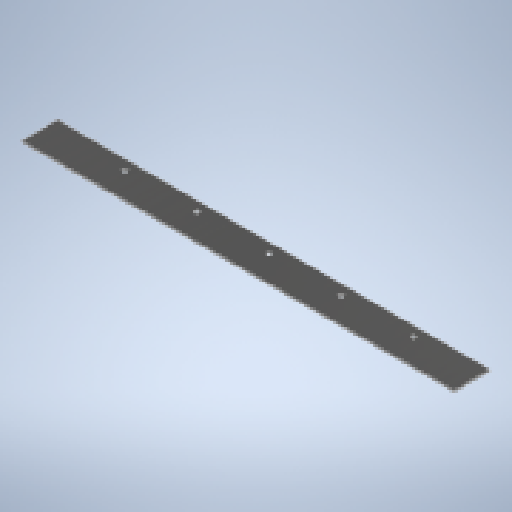
# Autodesk Inventor part: HCMUTE-CDT23-BTC-VND
Saved by Autodesk Inventor 2023 (Build 270158000, 158)
## iProperties
Created: 2023-11-27
Part Number: HCMUTE-CDT23-BTC-VND
Material: PMMA Plastic
Document SubType Name: Sheet Metal
Designer: havie
Density: 1.188 g/cm^3
Sheet Metal Rule: Default_mm
Appearance: Dark Gray
Author: havie
Autodesk Inventor part; units mm, degrees
ref_plane "YZ Plane" through (0, 0, 0) normal (1, 0, 0) x (0, 1, 0)
ref_plane "XZ Plane" through (0, 0, 0) normal (0, 1, 0) x (-1, 0, 0)
ref_plane "XY Plane" through (0, 0, 0) normal (0, 0, 1) x (1, 0, 0)
sketch "Sketch1" plane through (0, 0, 0) normal (0, 1, 0) x (-1, 0, 0)
  line L0 (-300, 25) -> (300, 25)
  line L1 (300, 25) -> (300, -25)
  line L2 (300, -25) -> (-300, -25)
  line L3 (-300, -25) -> (-300, 25)
  line L4 (-300, 25) -> (300, -25) construction
  line L5 (300, 25) -> (-300, -25) construction
  point P0 (0, 0)
  dimension "d0" = 600
  dimension "d1" = 50
  measures "d0" distance of L1.end L2.end
  measures "d1" distance of L2.end L0.start
extrude "Plate1" add sketch "Sketch1" along normal mid plane 2
sketch "Sketch2" plane through (0, -1, 0) normal (0, -1, 0) x (1, 0, 0)
  circle A0 centre (-192.5, -11) radius 2.5 projected
  circle A1 centre (-92.5, -11) radius 2.5 projected
  circle A2 centre (7.5, -11) radius 2.5 projected
  line L0 (300, 25) -> (-300, 25) projected
  line L1 (-300, 25) -> (-300, -25) projected
  line L2 (-300, -25) -> (300, -25) projected
  line L3 (300, -25) -> (300, 25) projected
  circle A3 centre (107.5, -11) radius 2.5 projected
  circle A4 centre (207.5, -11) radius 2.5 projected
  point P0 (0, 0)
  constraints: 5 coincident
hole "Hole1" at (-192.5, -1, -11) at (-92.5, -1, -11) at (7.5, -1, -11) at (107.5, -1, -11) at (207.5, -1, -11) direction (0, 1, 0) diameter 6 end through all
equation "\"d8\" = Thickness"
equation "\"d2\" = Thickness"
equation "\"BendRadius\" = Thickness"
equation "\"BendReliefWidth\" = Thickness"
equation "\"BendReliefDepth\" = 0.5 * Thickness"
equation "\"CornerReliefSize\" = 4 * Thickness"
equation "\"MinimumRemnant\" = 2 * Thickness"
equation "\"TransitionRadius\" = BendRadius"
equation "\"JacobiRadiusSize\" = BendRadius"
equation "\"GapSize\" = Thickness"
equation "\"Thickness\" = 2"
body "Solid1"
